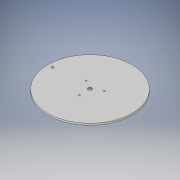
# Autodesk Inventor part: tourelle
Saved by Autodesk Inventor 2019 (Build 230136000, 136)
## iProperties
Created: 2018-05-17
Part Number: tourelle
Material: Générique
Document SubType Name: Modeling
Designer: Theo
Density: 1 g/cm^3
Appearance: Par défaut
Author: Theo
Autodesk Inventor part; units mm, degrees
ref_plane "YZ Plane" through (0, 0, 0) normal (1, 0, 0) x (0, 1, 0)
ref_plane "XZ Plane" through (0, 0, 0) normal (0, 1, 0) x (-1, 0, 0)
ref_plane "XY Plane" through (0, 0, 0) normal (0, 0, 1) x (1, 0, 0)
sketch "Esquisse1" plane through (0, 0, 0) normal (0, 1, 0) x (-1, 0, 0)
  circle A0 centre (0, 0) radius 5 construction
  circle A1 centre (0, 0) radius 120
  dimension "d0" = 10
  dimension "d39" = 240
  constraints: 2 centre point, 2 coincident
  measures "d0" diameter of A0
  measures "d39" diameter of A1
extrude "Extrusion1" add sketch "Esquisse1" along normal blind 5
sketch "Esquisse2" plane through (0, 5, 0) normal (0, 1, 0) x (1, 0, 0)
  circle A0 centre (0, 0) radius 5
  dimension "d5" = 10
  constraints: 1 centre point, 1 coincident
  measures "d5" diameter of A0
extrude "Extrusion2" cut sketch "Esquisse2" against normal up to surface (5 mm away)
sketch "Esquisse3" plane through (0, 0, 0) normal (0, -1, 0) x (1, 0, 0)
  circle A0 centre (0, 0) radius 5 projected
  circle A1 centre (0, 0) radius 12.5
  dimension "d8" = 25
  constraints: 1 centre point, 1 coincident
  measures "d8" diameter of A1
extrude "Extrusion3" cut sketch "Esquisse3" against normal blind 2
chamfer "Chanfrein1" distance 0.5 angle 45 3 edges at (-12.5, 0, 0) (-5, 2, 0) (-5, 5, 0)
sketch "Esquisse4" plane through (0, 5, 0) normal (0, 1, 0) x (1, 0, 0)
  point P0 (0, 0)
  point P1 (0, -30)
  point P2 (25.9808, 15)
  point P3 (-25.9808, 15)
  dimension "d14" = 30
  dimension "d17" = 360
  constraints: 1 vertical alignment, 4 other
  measures "d14" distance of point (0, -30) point (0, 0)
hole "Perçage1" at (0, 5, 30) at (25.9808, 5, -15) at (-25.9808, 5, -15) direction (0, -1, 0) diameter 4.2 depth 3 tip angle 118
sketch "Esquisse6" plane through (0, 5, 0) normal (0, 1, 0) x (1, 0, 0)
  circle A0 centre (-107, 0) radius 3
  point P0 (0, 0)
  dimension "d42" = 6
  dimension "d43" = 107
  constraints: 1 centre point, 1 horizontal alignment
  measures "d42" diameter of A0
  measures "d43" distance of A0.centre point (0, 0)
extrude "Extrusion5" cut sketch "Esquisse6" against normal up to surface (5 mm away)
